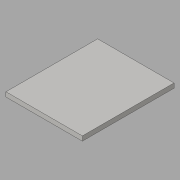
# Autodesk Inventor part: c1g
Saved by Autodesk Inventor 2016 (Build 200138000, 138)
## iProperties
Created: 2015-10-11
Part Number: c1g
Material: Generic
Document SubType Name: Modeling
Designer: daniel
Density: 1 g/cm^3
Appearance: Default
Author: daniel
Autodesk Inventor part; units mm, degrees
ref_plane "YZ Plane" through (0, 0, 0) normal (1, 0, 0) x (0, 1, 0)
ref_plane "XZ Plane" through (0, 0, 0) normal (0, 1, 0) x (-1, 0, 0)
ref_plane "XY Plane" through (0, 0, 0) normal (0, 0, 1) x (1, 0, 0)
derived "base.ipt"
sketch "sketch_projected_dwg" plane through (0, 0, 0) normal (0, 0, 1) x (1, 0, 0)
  line L0 (1992.3758, -140.1528) -> (1992.3758, -170.1528)
  line L1 (1992.3758, -170.1528) -> (2025.8085, -170.1528)
  line L2 (2025.8085, -170.1528) -> (2025.8085, -140.1528)
  line L3 (2025.8085, -140.1528) -> (2029.0921, -140.1528)
  line L4 (2029.0921, -140.1528) -> (2029.0921, -173.5311)
  line L5 (2029.0921, -173.5311) -> (2049.0921, -173.5311)
  line L6 (2049.0921, -173.5311) -> (2049.0921, -170.1528)
  line L7 (2049.0921, -170.1528) -> (2059.0921, -170.1528)
  line L8 (2059.0921, -170.1528) -> (2059.0921, -110.1528)
  line L9 (2059.0921, -110.1528) -> (2049.0921, -110.1528)
  line L10 (2049.0921, -110.1528) -> (2049.0921, -107.1528)
  line L11 (2049.0921, -107.1528) -> (2029.0921, -107.0583)
  line L12 (2029.0921, -107.0583) -> (2029.0921, -110.1528)
  line L13 (2029.0921, -110.1528) -> (1989.0921, -110.1528)
  line L14 (1989.0921, -110.1528) -> (1989.0921, -106.8691)
  line L15 (1989.0921, -106.8691) -> (1969.0921, -106.7746)
  line L16 (1969.0921, -106.7746) -> (1969.0921, -110.1528)
  line L17 (1969.0921, -110.1528) -> (1959.0921, -110.1528)
  line L18 (1959.0921, -110.1528) -> (1959.0921, -170.1528)
  line L19 (1959.0921, -170.1528) -> (1969.0921, -170.1528)
  line L20 (1969.0921, -170.1528) -> (1969.0921, -173.5311)
  line L21 (1969.0921, -173.5311) -> (1989.0921, -173.5311)
  line L22 (1989.0921, -173.5311) -> (1989.0921, -140.1528)
  line L23 (1989.0921, -140.1528) -> (1992.3758, -140.1528)
  line L24 (1992.3758, -228.8911) -> (1992.3758, -258.8911)
  line L25 (1992.3758, -258.8911) -> (1989.0921, -258.8911)
  line L26 (1989.0921, -258.8911) -> (1989.0921, -228.8911)
  line L27 (1989.0921, -228.8911) -> (1959.0921, -228.8911)
  line L28 (1959.0921, -228.8911) -> (1959.0921, -288.8911)
  line L29 (1959.0921, -288.8911) -> (2059.0921, -288.8911)
  line L30 (2059.0921, -288.8911) -> (2059.0921, -228.8911)
  line L31 (2059.0921, -228.8911) -> (2029.0921, -228.8911)
  line L32 (2029.0921, -228.8911) -> (2029.0921, -258.8911)
  line L33 (2029.0921, -258.8911) -> (2025.8085, -258.8911)
  line L34 (2025.8085, -258.8911) -> (2025.8085, -228.8911)
  line L35 (2025.8085, -228.8911) -> (1992.3758, -228.8911)
  circle A0 centre (2039.0921, -262.8911) radius 6
  circle A1 centre (2009.0921, -262.8911) radius 4.7571
  circle A2 centre (1979.0921, -262.8911) radius 6
  line L36 (2365.3683, 1.7867) -> (2365.3683, -98.2133)
  line L37 (2471.3683, 1.7867) -> (2471.3683, -98.2133)
  line L38 (2371.3683, -263.5692) -> (2371.3683, -363.5692)
  line L39 (2465.3683, -263.5692) -> (2465.3683, -363.5692)
  line L40 (2311.3683, -263.5692) -> (2371.3683, -263.5692)
  line L41 (2371.3683, -263.5692) -> (2418.3683, -263.5692)
  line L42 (2418.3683, -263.5692) -> (2465.3683, -263.5692)
  line L43 (2465.3683, -263.5692) -> (2525.3683, -263.5692)
  line L44 (2525.3683, -263.5692) -> (2525.3683, -333.5692)
  line L45 (2525.3683, -333.5692) -> (2495.3683, -363.5692)
  line L46 (2495.3683, -363.5692) -> (2341.3683, -363.5692)
  line L47 (2341.3683, -363.5692) -> (2311.3683, -333.5692)
  line L48 (2311.3683, -333.5692) -> (2311.3683, -263.5692)
  line L49 (2398.3683, -278.5692) -> (2401.3683, -278.5692)
  line L50 (2401.3683, -278.5692) -> (2401.3683, -298.5692)
  line L51 (2401.3683, -298.5692) -> (2398.3683, -298.5692)
  line L52 (2398.3683, -298.5692) -> (2398.3683, -278.5692)
  line L53 (2435.3683, -278.5692) -> (2438.3683, -278.5692)
  line L54 (2438.3683, -278.5692) -> (2438.3683, -298.5692)
  line L55 (2438.3683, -298.5692) -> (2435.3683, -298.5692)
  line L56 (2435.3683, -298.5692) -> (2435.3683, -278.5692)
  line L57 (2435.3683, -328.5692) -> (2438.3683, -328.5692)
  line L58 (2438.3683, -328.5692) -> (2438.3683, -348.5692)
  line L59 (2438.3683, -348.5692) -> (2435.3683, -348.5692)
  line L60 (2435.3683, -348.5692) -> (2435.3683, -328.5692)
  line L61 (2398.3683, -328.5692) -> (2401.3683, -328.5692)
  line L62 (2401.3683, -328.5692) -> (2401.3683, -348.5692)
  line L63 (2401.3683, -348.5692) -> (2398.3683, -348.5692)
  line L64 (2398.3683, -348.5692) -> (2398.3683, -328.5692)
  line L65 (2398.3683, -63.2133) -> (2401.3683, -63.2133)
  line L66 (2401.3683, -63.2133) -> (2401.3683, -83.2133)
  line L67 (2401.3683, -83.2133) -> (2398.3683, -83.2133)
  line L68 (2398.3683, -83.2133) -> (2398.3683, -63.2133)
  line L69 (2368.3683, -63.2133) -> (2371.3683, -63.2133)
  line L70 (2371.3683, -63.2133) -> (2371.3683, -83.2133)
  line L71 (2371.3683, -83.2133) -> (2368.3683, -83.2133)
  line L72 (2368.3683, -83.2133) -> (2368.3683, -63.2133)
  line L73 (2368.3683, -13.2133) -> (2371.3683, -13.2133)
  line L74 (2371.3683, -13.2133) -> (2371.3683, -33.2133)
  line L75 (2371.3683, -33.2133) -> (2368.3683, -33.2133)
  line L76 (2368.3683, -33.2133) -> (2368.3683, -13.2133)
  line L77 (2398.3683, -13.2133) -> (2401.3683, -13.2133)
  line L78 (2401.3683, -13.2133) -> (2401.3683, -33.2133)
  line L79 (2401.3683, -33.2133) -> (2398.3683, -33.2133)
  line L80 (2398.3683, -33.2133) -> (2398.3683, -13.2133)
  line L81 (2435.3683, -13.2133) -> (2438.3683, -13.2133)
  line L82 (2438.3683, -13.2133) -> (2438.3683, -33.2133)
  line L83 (2438.3683, -33.2133) -> (2435.3683, -33.2133)
  line L84 (2435.3683, -33.2133) -> (2435.3683, -13.2133)
  line L85 (2465.3683, -13.2133) -> (2468.3683, -13.2133)
  line L86 (2468.3683, -13.2133) -> (2468.3683, -33.2133)
  line L87 (2468.3683, -33.2133) -> (2465.3683, -33.2133)
  line L88 (2465.3683, -33.2133) -> (2465.3683, -13.2133)
  line L89 (2465.3683, -63.2133) -> (2468.3683, -63.2133)
  line L90 (2468.3683, -63.2133) -> (2468.3683, -83.2133)
  line L91 (2468.3683, -83.2133) -> (2465.3683, -83.2133)
  line L92 (2465.3683, -83.2133) -> (2465.3683, -63.2133)
  line L93 (2435.3683, -63.2133) -> (2438.3683, -63.2133)
  line L94 (2438.3683, -63.2133) -> (2438.3683, -83.2133)
  line L95 (2438.3683, -83.2133) -> (2435.3683, -83.2133)
  line L96 (2435.3683, -83.2133) -> (2435.3683, -63.2133)
  line L97 (2518.3683, -98.2133) -> (2468.3683, -98.2133)
  line L98 (2468.3683, 61.7867) -> (2518.3683, 61.7867)
  line L99 (2518.3683, 61.7867) -> (2518.3683, 1.7867)
  line L100 (2518.3683, 1.7867) -> (2594.3683, 1.7867)
  line L101 (2594.3683, 1.7867) -> (2594.3683, -13.2133)
  line L102 (2594.3683, -13.2133) -> (2597.3683, -13.2133)
  line L103 (2597.3683, -13.2133) -> (2597.3683, -33.2133)
  line L104 (2597.3683, -33.2133) -> (2594.3683, -33.2133)
  line L105 (2594.3683, -33.2133) -> (2594.3683, -48.2133)
  line L106 (2594.3683, -48.2133) -> (2594.3683, -63.2133)
  line L107 (2594.3683, -63.2133) -> (2597.3683, -63.2133)
  line L108 (2597.3683, -63.2133) -> (2597.3683, -83.2133)
  line L109 (2597.3683, -83.2133) -> (2594.3683, -83.2133)
  line L110 (2594.3683, -83.2133) -> (2594.3683, -98.2133)
  line L111 (2594.3683, -98.2133) -> (2518.3683, -98.2133)
  line L112 (2518.3683, -98.2133) -> (2518.3683, -158.2133)
  line L113 (2518.3683, -158.2133) -> (2391.6842, -158.2133)
  line L114 (2531.3683, 1.7867) -> (2531.3683, -98.2133)
  line L115 (2534.3683, 1.7867) -> (2534.3683, -98.2133)
  line L116 (2368.3683, -158.2133) -> (2368.3683, -98.2133)
  line L117 (2368.3683, -98.2133) -> (2468.3683, -98.2133)
  line L118 (2468.3683, -98.2133) -> (2468.3683, -158.2133)
  circle A3 centre (2448.3683, -124.2133) radius 6
  circle A4 centre (2426.6172, -119.4508) radius 1.5
  circle A5 centre (2418.3683, -124.2133) radius 6.35
  circle A6 centre (2410.1194, -119.4508) radius 1.5
  circle A7 centre (2418.3683, -133.7383) radius 1.5
  circle A8 centre (2388.3683, -124.2133) radius 6
  line L119 (2368.3683, -158.2133) -> (2418.3683, -158.2133)
  line L120 (2418.3683, -158.2133) -> (2468.3683, -158.2133)
  line L121 (2391.6842, -158.2133) -> (2318.3683, -158.2133)
  line L122 (2318.3683, -158.2133) -> (2318.3683, -98.2133)
  line L123 (2318.3683, -98.2133) -> (2242.3683, -98.2133)
  line L124 (2242.3683, -98.2133) -> (2242.3683, -83.2133)
  line L125 (2242.3683, -83.2133) -> (2239.3683, -83.2133)
  line L126 (2239.3683, -83.2133) -> (2239.3683, -63.2133)
  line L127 (2239.3683, -63.2133) -> (2242.3683, -63.2133)
  line L128 (2242.3683, -63.2133) -> (2242.3683, -48.2133)
  line L129 (2242.3683, -48.2133) -> (2242.3683, -33.2133)
  line L130 (2242.3683, -33.2133) -> (2239.3683, -33.2133)
  line L131 (2239.3683, -33.2133) -> (2239.3683, -13.2133)
  line L132 (2239.3683, -13.2133) -> (2242.3683, -13.2133)
  line L133 (2242.3683, -13.2133) -> (2242.3683, 1.7867)
  line L134 (2242.3683, 1.7867) -> (2318.3683, 1.7867)
  line L135 (2318.3683, 1.7867) -> (2318.3683, 61.7867)
  line L136 (2318.3683, -98.2133) -> (2368.3683, -98.2133)
  line L137 (2305.3683, 1.7867) -> (2305.3683, -98.2133)
  line L138 (2302.3683, 1.7867) -> (2302.3683, -98.2133)
  line L139 (2318.3683, 61.7867) -> (2368.3683, 61.7867)
  line L140 (2368.3683, 61.7867) -> (2418.3683, 61.7867)
  line L141 (2418.3683, 61.7867) -> (2468.3683, 61.7867)
  line L142 (2368.3683, 61.7867) -> (2368.3683, 1.7867)
  line L143 (2368.3683, 1.7867) -> (2468.3683, 1.7867)
  line L144 (2468.3683, 1.7867) -> (2468.3683, 61.7867)
  circle A9 centre (2388.3683, 27.7867) radius 6
  circle A10 centre (2418.3683, 27.7867) radius 4.5
  circle A11 centre (2448.3683, 27.7867) radius 6
  line L145 (2518.3683, 1.7867) -> (2468.3683, 1.7867)
  line L146 (2318.3683, 1.7867) -> (2368.3683, 1.7867)
  line L147 (1486.5912, 319.5306) -> (1298.5912, 319.5306)
  line L148 (1298.5912, 319.5306) -> (1298.5912, 259.5306)
  line L149 (1298.5912, 259.5306) -> (1486.5912, 259.5306)
  line L150 (1486.5912, 259.5306) -> (1594.5912, 259.5306)
  line L151 (1594.5912, 259.5306) -> (1782.5912, 259.5306)
  line L152 (1782.5912, 259.5306) -> (1782.5912, 319.5306)
  line L153 (1782.5912, 319.5306) -> (1594.5912, 319.5306)
  line L154 (1594.5912, 319.5306) -> (1486.5912, 319.5306)
  line L155 (1594.5912, 319.5306) -> (1594.5912, 259.5306)
  circle A12 centre (1570.5912, 294.5306) radius 5
  circle A13 centre (1556.0912, 310.0306) radius 1.5
  circle A14 centre (1556.0912, 279.0306) radius 1.5
  circle A15 centre (1540.5912, 294.5306) radius 4.5
  circle A16 centre (1510.5912, 294.5306) radius 5
  circle A17 centre (1525.0912, 279.0306) radius 1.5
  circle A18 centre (1525.0912, 310.0306) radius 1.5
  line L156 (1486.5912, 319.5306) -> (1486.5912, 259.5306)
  line L157 (1486.5912, 198.0466) -> (1486.5912, 138.0466)
  line L158 (1486.5912, 198.0466) -> (1298.5912, 198.0466)
  line L159 (1298.5912, 198.0466) -> (1298.5912, 138.0466)
  line L160 (1298.5912, 138.0466) -> (1782.5912, 138.0466)
  line L161 (1782.5912, 138.0466) -> (1782.5912, 198.0466)
  line L162 (1782.5912, 198.0466) -> (1594.5912, 198.0466)
  line L163 (1594.5912, 198.0466) -> (1486.5912, 198.0466)
  line L164 (1594.5912, 198.0466) -> (1594.5912, 138.0466)
  circle A19 centre (1570.5912, 173.0466) radius 5
  circle A20 centre (1540.5912, 173.0466) radius 4.5
  circle A21 centre (1510.5912, 173.0466) radius 5
  line L165 (1565.5912, 43.4562) -> (1515.5912, 43.4562)
  line L166 (1515.5912, 43.4562) -> (1515.5912, 37.4562)
  line L167 (1515.5912, 37.4562) -> (1515.5912, 18.4562)
  line L168 (1515.5912, 18.4562) -> (1565.5912, 18.4562)
  line L169 (1565.5912, 18.4562) -> (1565.5912, 37.4562)
  line L170 (1565.5912, 37.4562) -> (1565.5912, 43.4562)
  line L171 (1486.5912, 40.4562) -> (1515.5912, 40.4562)
  line L172 (1461.5912, 100.4562) -> (1461.5912, 40.4562)
  line L173 (1461.5912, 40.4562) -> (1486.5912, 40.4562)
  line L174 (1486.5912, 100.4562) -> (1486.5912, 40.4562)
  line L175 (1461.5912, 100.4562) -> (1486.5912, 100.4562)
  line L176 (1486.5912, 100.4562) -> (1594.5912, 100.4562)
  circle A22 centre (1510.5912, 75.4562) radius 5
  circle A23 centre (1540.5912, 75.4562) radius 4.5
  circle A24 centre (1570.5912, 75.4562) radius 5
  line L177 (1594.5912, 100.4562) -> (1594.5912, 40.4562)
  line L178 (1594.5912, 40.4562) -> (1565.5912, 40.4562)
  line L179 (1594.5912, 40.4562) -> (1619.5912, 40.4562)
  line L180 (1619.5912, 100.4562) -> (1619.5912, 40.4562)
  line L181 (1594.5912, 100.4562) -> (1619.5912, 100.4562)
  line L182 (1486.5912, -242.3994) -> (1594.5912, -242.3994)
  line L183 (1486.5912, -242.3994) -> (1486.5912, -302.3994)
  circle A25 centre (1525.0912, -251.8994) radius 1.5
  line L184 (1594.5912, -242.3994) -> (1594.5912, -302.3994)
  circle A26 centre (1570.5912, -267.3994) radius 5
  circle A27 centre (1556.0912, -251.8994) radius 1.5
  circle A28 centre (1556.0912, -282.8994) radius 1.5
  circle A29 centre (1525.0912, -282.8994) radius 1.5
  circle A30 centre (1540.5912, -267.3994) radius 11
  circle A31 centre (1510.5912, -267.3994) radius 5
  line L185 (1486.5912, -302.3994) -> (1515.5912, -302.3994)
  line L186 (1515.5912, -299.3994) -> (1515.5912, -305.3994)
  line L187 (1515.5912, -305.3994) -> (1515.5912, -324.3994)
  line L188 (1515.5912, -324.3994) -> (1565.5912, -324.3994)
  line L189 (1565.5912, -324.3994) -> (1565.5912, -305.3994)
  line L190 (1565.5912, -305.3994) -> (1565.5912, -299.3994)
  line L191 (1565.5912, -299.3994) -> (1515.5912, -299.3994)
  line L192 (1594.5912, -302.3994) -> (1565.5912, -302.3994)
  line L193 (592.8683, 248.864) -> (592.8683, 495.864)
  line L194 (592.8683, 495.864) -> (532.8683, 495.864)
  line L195 (532.8683, 495.864) -> (532.8683, 317.864)
  line L196 (532.8683, 317.864) -> (529.8683, 317.864)
  line L197 (529.8683, 317.864) -> (529.8683, 397.864)
  line L198 (529.8683, 397.864) -> (479.8683, 397.864)
  line L199 (479.8683, 397.864) -> (479.8683, 317.864)
  line L200 (479.8683, 317.864) -> (473.8683, 317.864)
  line L201 (473.8683, 317.864) -> (473.8683, 417.864)
  line L202 (473.8683, 417.864) -> (97.8683, 417.864)
  line L203 (97.8683, 417.864) -> (97.8683, 317.864)
  line L204 (97.8683, 317.864) -> (91.8683, 317.864)
  line L205 (91.8683, 317.864) -> (91.8683, 397.864)
  line L206 (91.8683, 397.864) -> (41.8683, 397.864)
  line L207 (41.8683, 397.864) -> (41.8683, 317.864)
  line L208 (41.8683, 317.864) -> (38.8683, 317.864)
  line L209 (38.8683, 317.864) -> (38.8683, 495.864)
  line L210 (38.8683, 495.864) -> (-21.1317, 495.864)
  line L211 (-21.1317, 495.864) -> (-21.1317, 248.864)
  line L212 (479.8683, 377.864) -> (529.8683, 377.864)
  line L213 (479.8683, 374.864) -> (529.8683, 374.864)
  line L214 (97.8683, 374.864) -> (473.8683, 374.864)
  line L215 (473.8683, 377.864) -> (97.8683, 377.864)
  line L216 (529.8683, 317.864) -> (479.8683, 317.864)
  line L217 (473.8683, 317.864) -> (97.8683, 317.864)
  line L218 (532.8683, 311.864) -> (38.8683, 311.864)
  line L219 (532.8683, 317.864) -> (532.8683, 311.864)
  line L220 (532.8683, 311.864) -> (532.8683, 251.864)
  line L221 (592.8683, 248.864) -> (532.8683, 248.864)
  line L222 (532.8683, 134.864) -> (532.8683, 248.864)
  line L223 (38.8683, 251.864) -> (532.8683, 251.864)
  line L224 (532.8683, 248.864) -> (532.8683, 251.864)
  line L225 (592.8683, 248.864) -> (592.8683, 134.864)
  circle A32 centre (567.8683, 221.864) radius 5
  circle A33 centre (567.8683, 161.864) radius 5
  line L226 (592.8683, 134.864) -> (532.8683, 134.864)
  line L227 (478.2659, 201.8775) -> (478.2659, 191.8909)
  line L228 (478.2659, 191.864) -> (478.2659, 181.8775)
  line L229 (54.3241, 181.8775) -> (478.2659, 181.8775)
  line L230 (54.3241, 201.8775) -> (478.2659, 201.8775)
  line L231 (38.8683, 131.864) -> (532.8683, 131.864)
  line L232 (532.8683, 134.864) -> (532.8683, 131.864)
  line L233 (38.8683, 248.864) -> (38.8683, 134.864)
  line L234 (38.8683, 134.864) -> (-21.1317, 134.864)
  line L235 (38.8683, 134.864) -> (38.8683, 131.864)
  line L236 (38.8683, 248.864) -> (38.8683, 251.864)
  line L237 (-21.1317, 248.864) -> (38.8683, 248.864)
  line L238 (-21.1317, 248.864) -> (-21.1317, 134.864)
  circle A34 centre (3.8683, 217.5276) radius 5
  circle A35 centre (3.8683, 155.5276) radius 5
  line L239 (38.8683, 317.864) -> (38.8683, 305.864)
  line L240 (38.8683, 305.864) -> (38.8683, 251.864)
  line L241 (41.8683, 317.864) -> (91.8683, 317.864)
  line L242 (91.8683, 374.864) -> (41.8683, 374.864)
  line L243 (91.8683, 377.864) -> (41.8683, 377.864)
  line L244 (54.3241, 201.8775) -> (54.3241, 181.8775)
  point P0 (0, 0)
extrude "Extrusion1" add sketch "sketch_projected_dwg" along normal blind 3 contours L136 L116 L121 L122
equation "\"d1\" = material_thickness"
equation "\"material_thickness\" = 3"
body "Solid1"
